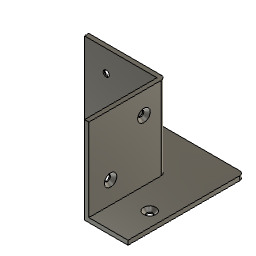
Bottom_Table_Leg_Mount_x4 (Autodesk Fusion 360 design; units mm, degrees)
Autodesk Fusion 360 part; units mm, degrees
sketch "Sketch1" plane through (0, 0, 0) normal (0, 0, 1) x (1, 0, 0)
  line L0 (-30.479, 50.2485) -> (19.521, 50.2485)
  line L1 (19.521, 50.2485) -> (19.521, 0.2485)
  line L2 (19.521, 0.2485) -> (49.521, 0.2485)
  line L3 (-30.479, 50.2485) -> (-30.479, 80.2485)
  line L4 (-30.479, 80.2485) -> (49.521, 80.2485)
  line L5 (49.521, 80.2485) -> (49.521, 0.2485)
  line L6 (19.521, 0.2485) -> (22.521, 0.2485)
  line L7 (-30.479, 50.2485) -> (-30.479, 53.2485)
  line L8 (-30.479, 53.2485) -> (22.521, 53.2485)
  line L9 (22.521, 53.2485) -> (22.521, 0.2485)
  dimension "d1" = 50
  dimension "d2" = 50
  dimension "d3" = 30
  dimension "d4" = 30
  dimension "d5" = 80
  dimension "d6" = 3
  dimension "d7" = 3
  dimension "d8" = 53
  constraint horizontal L0
  constraint perpendicular L0 L1
  constraint perpendicular L1 L2
  constraint perpendicular L0 L3
  constraint perpendicular L3 L4
  constraint perpendicular L1 L6
  constraint perpendicular L0 L7
  constraint perpendicular L1 L8
  measures "d1" distance of L0.start L0.end
  measures "d2" distance of L0.end L1.end
  measures "d3" distance of L1.end L2.end
  measures "d4" distance of L0.start L3.end
  measures "d5" distance of L3.end L4.end
  measures "d6" distance of L1.end L6.end
  measures "d7" distance of L0.start L7.end
  measures "d8" distance of L7.end L8.end
extrude "Extrude1" add sketch "Sketch1" along normal blind 3 makes body 1
extrude "Extrude2" add sketch "Sketch1" along normal blind 60 separate body contours L0 L1 L2 L3 L6 L7 L8 L9 makes body 2
combine "Combine1" operation add target body 2 tool bodies 1
sketch "Sketch2" plane through (0, 0, 3) normal (0, 0, 1) x (-1, 0, 0)
  line L0 (30.479, -53.2485) -> (-22.521, -53.2485)
  line L1 (-22.521, -53.2485) -> (-22.521, -0.2485)
  line L2 (-22.521, -0.2485) -> (-49.521, -0.2485)
  line L3 (-49.521, -0.2485) -> (-49.521, -80.2485)
  line L4 (-49.521, -80.2485) -> (30.479, -80.2485)
  line L5 (30.479, -80.2485) -> (30.479, -53.2485)
  line L6 (-49.521, -0.2485) -> (-39.521, -0.2485)
  line L7 (-39.521, -0.2485) -> (-39.521, -25.2485)
  line L8 (30.479, -80.2485) -> (30.479, -70.2485)
  line L9 (30.479, -70.2485) -> (5.479, -70.2485)
  dimension "d13" = 10
  dimension "d14" = 25
  dimension "d15" = 10
  dimension "d16" = 25
  constraint coincident L2.end L3.start
  constraint perpendicular L3 L6
  constraint perpendicular L2 L7
  constraint coincident L4.end L5.start
  constraint perpendicular L4 L8
  constraint perpendicular L5 L9
  measures "d13" distance of L2.end L6.end
  measures "d14" distance of L6.end L7.end
  measures "d15" distance of L4.end L8.end
  measures "d16" distance of L8.end L9.end
hole "Hole1" at (39.521, 25.2485, 3) at (-5.479, 70.2485, 3) direction (0, 0, -1) diameter 4.2 end through all countersink diameter 8.6 countersink angle 90 bodies 2
sketch "Sketch3" plane through (22.521, 0, 0) normal (1, 0, 0) x (0, 1, 0)
  line L0 (0.2485, 3) -> (53.2485, 3)
  line L1 (53.2485, 3) -> (53.2485, 60)
  line L2 (53.2485, 60) -> (0.2485, 60)
  line L3 (0.2485, 60) -> (0.2485, 3)
  line L4 (0.2485, 3) -> (0.2485, 18)
  line L5 (0.2485, 18) -> (15.2485, 18)
  line L6 (53.2485, 60) -> (53.2485, 45)
  line L7 (53.2485, 45) -> (38.2485, 45)
  dimension "d22" = 15
  dimension "d23" = 15
  dimension "d24" = 15
  dimension "d25" = 15
  constraint coincident L0.start L3.end
  constraint perpendicular L0 L4
  constraint perpendicular L4 L5
  constraint coincident L1.end L2.start
  constraint perpendicular L2 L6
  constraint perpendicular L6 L7
  measures "d22" distance of L0.start L4.end
  measures "d23" distance of L4.end L5.end
  measures "d24" distance of L1.end L6.end
  measures "d25" distance of L6.end L7.end
hole "Hole2" at (22.521, 15.2485, 18) at (22.521, 38.2485, 45) direction (-1, 0, 0) diameter 4.2 end through all countersink diameter 8.6 countersink angle 90 bodies 2
sketch "Sketch4" plane through (0, 53.2485, 0) normal (0, 1, 0) x (-1, 0, 0)
  line L0 (-22.521, 3) -> (30.479, 3)
  line L1 (30.479, 3) -> (30.479, 60)
  line L2 (30.479, 60) -> (-22.521, 60)
  line L3 (-22.521, 60) -> (-22.521, 3)
  line L4 (-22.521, 3) -> (-22.521, 18)
  line L5 (-22.521, 18) -> (-7.521, 18)
  line L6 (30.479, 60) -> (30.479, 45)
  line L7 (30.479, 45) -> (15.479, 45)
  dimension "d31" = 15
  dimension "d32" = 15
  dimension "d33" = 15
  dimension "d34" = 15
  constraint coincident L0.start L3.end
  constraint perpendicular L0 L4
  constraint perpendicular L3 L5
  constraint coincident L1.end L2.start
  constraint perpendicular L2 L6
  constraint perpendicular L6 L7
  measures "d31" distance of L0.start L4.end
  measures "d32" distance of L4.end L5.end
  measures "d33" distance of L1.end L6.end
  measures "d34" distance of L6.end L7.end
hole "Hole3" at (-15.479, 53.2485, 45) at (7.521, 53.2485, 18) direction (0, -1, 0) diameter 4.2 end through all countersink diameter 8.6 countersink angle 90 bodies 2
fillet "Fillet1" radius 3 2 edges at (22.521, 53.2485, 31.5) (49.521, 80.2485, 1.5) on bodies 2
